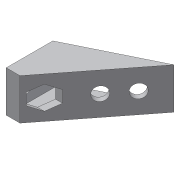
# Autodesk Inventor part: Befestigung
Saved by Autodesk Inventor 2013 (Build 170138000, 138)
## iProperties
Created: 2013-07-03
Part Number: Befestigung
Material: Allgemein
Document SubType Name: Modeling
Designer: Harald
Density: 1 g/cm^3
Author: Harald
Autodesk Inventor part; units mm, degrees
ref_plane "YZ Plane" through (0, 0, 0) normal (1, 0, 0) x (0, 1, 0)
ref_plane "XZ Plane" through (0, 0, 0) normal (0, 1, 0) x (-1, 0, 0)
ref_plane "XY Plane" through (0, 0, 0) normal (0, 0, 1) x (1, 0, 0)
sketch "Skizze1" plane through (0, 0, 0) normal (0, 0, 1) x (1, 0, 0)
  line L0 (0, 0) -> (0, 17)
  line L1 (0, 0) -> (40, 0) construction
  line L2 (0, 0) -> (5, 0)
  line L3 (5, 0) -> (29.6265, 31.5204)
  line L4 (29.6265, 31.5204) -> (0, 17)
  dimension "d0" = 17
  dimension "d46" = 5
  dimension "d48" = 40
  constraints: 10 end point, 1 horizontal, 1 point on line, 1 vertical
  measures "d0" distance of L0.start L0.end
  measures "d46" distance of L0.start L2.end
  measures "d48" distance of L2.end L3.end
extrude "Extrusion1" add sketch "Skizze1" along normal blind 15
hole "Bohrung1" at (0, 5, 7.5) direction (1, 0, 0) diameter 5 end through all
shell "Wandstärke3" thickness 2 removed faces 2 at (9.8755, 21.8401, 5) at (3.6198, 7.5, 7.5084)
sketch "Skizze5" plane through (2, 2, 2) normal (1, 0, 0) x (0, 0, -1)
  circle A0 centre (-5.5, 3) radius 2.5 projected
  line L0 (-3.35, -0.7239) -> (-7.65, -0.7239)
  line L1 (-7.65, -0.7239) -> (-9.8, 3)
  line L2 (-9.8, 3) -> (-7.65, 6.7239)
  line L3 (-7.65, 6.7239) -> (-3.35, 6.7239)
  line L4 (-3.35, 6.7239) -> (-1.2, 3)
  line L5 (-1.2, 3) -> (-3.35, -0.7239)
  point P0 (2, -2)
  dimension "d71" = 4.3
  constraints: 12 end point, 1 coincident, 1 horizontal, 13 other
  measures "d71" distance of L4.end A0.centre
extrude "Extrusion4" cut sketch "Skizze5" along normal blind 10
hole "Bohrung6" at (22.4352, 25.5645, 7.5) direction (0.7880108, -0.6156615, 0) diameter 5 end through all
hole "Bohrung7" at (16.2786, 17.6844, 7.5) direction (0.7880108, -0.6156615, 0) diameter 5 end through all
